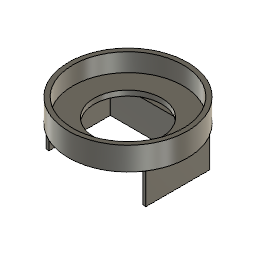
229d907d-bee8-423c-b9df-8a4b31d83d24 (Autodesk Fusion 360 design; units mm, degrees)
part number: 2026-05-18-17-01-56-091
Autodesk Fusion 360 part; units mm, degrees
sketch "スケッチ1" plane through (0, 0, 0) normal (0, 0, 1) x (1, 0, 0)
  circle A0 centre (0, 0) radius 23
  circle A1 centre (0, 0) radius 21.25
  dimension "d1" = 46
  dimension "d2" = 42.5
  constraint coincident A0.centre A1.centre
  constraint concentric A0 A1
  measures "d1" diameter of A0
  measures "d2" diameter of A1
extrude "押し出し1" add sketch "スケッチ1" along normal blind 2 contours A1
extrude "押し出し2" add sketch "スケッチ1" along normal blind 9
sketch "スケッチ2" plane through (0, 0, 0) normal (0, 0, -1) x (1, 0, 0)
  circle A0 centre (0, 0) radius 23
  circle A1 centre (0, 0) radius 13
  dimension "d7" = 26
  constraint concentric A0 A1
  measures "d7" diameter of A1
extrude "押し出し3" cut sketch "スケッチ2" against normal blind 3 contours A1
sketch "スケッチ3" plane through (0, 0, 0) normal (0, 0, -1) x (1, 0, 0)
  circle A0 centre (0, 0) radius 13
  circle A1 centre (0, 0) radius 23
  line L0 (18.1, -11.26) -> (-18.1, -11.26)
  line L1 (-18.1, -11.26) -> (-18.1, 14.3567)
  line L2 (-18.1, 14.3567) -> (18.1, 14.3567)
  line L3 (18.1, 14.3567) -> (18.1, -11.26)
  line L4 (19.3, -12.3) -> (-19.3, -12.3)
  line L5 (-19.3, -12.3) -> (-19.3, 12.4)
  line L6 (-19.3, 12.4) -> (19.3, 12.4)
  line L7 (19.3, 12.4) -> (19.3, -12.3)
  dimension "d10" = 11.26
  dimension "d11" = 18.1
  dimension "d12" = 18.1
  dimension "d13" = 12.3
  dimension "d14" = 19.3
  dimension "d15" = 19.3
  dimension "d16" = 12.4
  constraint horizontal L0
  constraint vertical L1
  constraint horizontal L2
  constraint vertical L3
  constraint horizontal L4
  constraint vertical L5
  constraint horizontal L6
  constraint vertical L7
  measures "d10" distance of A0.centre L0
  measures "d11" distance of A0.centre L3
  measures "d12" distance of A0.centre L1
  measures "d13" distance of A0.centre L4
  measures "d14" distance of A0.centre L7
  measures "d15" distance of A0.centre L5
  measures "d16" distance of A0.centre L6
extrude "押し出し4" add sketch "スケッチ3" along normal blind 12 contours A0 L0 L3 L4 L6 L7 | A0 L0 L4 | A0 L0 L1 L4 L5 L6
sketch "スケッチ4" plane through (0, 0, 0) normal (0, 0, 1) x (-1, 0, 0)
  arc A0 (4.2083, -12.3) -> (6.4971, -11.26) centre (0, 0) ccw
  line L0 (6.4971, -11.26) -> (-6.4971, -11.26)
  arc A1 (-6.4971, -11.26) -> (-4.2083, -12.3) centre (0, 0) ccw
  line L1 (-4.2083, -12.3) -> (4.2083, -12.3)
  line L2 (8.6335, -10.0758) -> (-7.7138, -10.0758)
  line L3 (-7.7138, -10.0758) -> (-7.7138, -15.2171)
  line L4 (-7.7138, -15.2171) -> (8.6335, -15.2171)
  line L5 (8.6335, -15.2171) -> (8.6335, -10.0758)
  circle A2 centre (0, 0) radius 13
  circle A3 centre (0, 0) radius 14
  line L6 (9.1438, -11.26) -> (-8.6053, -11.26)
  dimension "d19" = 26
  dimension "d20" = 28
  constraint horizontal L2
  constraint vertical L3
  constraint horizontal L4
  constraint vertical L5
  constraint concentric A0 A2
  constraint coincident A0.end A2
  constraint coincident A0.centre A1.centre
  constraint perpendicular L3 L6
  measures "d19" diameter of A2
  measures "d20" diameter of A3
extrude "押し出し5" add sketch "スケッチ4" against normal blind 2 contours L1 A2 | A0 A1 L3 A2 A3 L6
